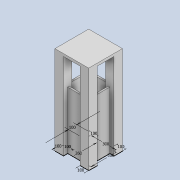
# Autodesk Inventor part: Part35
Saved by Autodesk Inventor 2021 (Build 250183000, 183)
## iProperties
Created: 2025-11-30
Part Number: Part35
Material: Generic
Document SubType Name: Modeling
Designer: huber
Density: 1 g/cm^3
Appearance: Default
Author: huber
Autodesk Inventor part; units mm, degrees
ref_plane "YZ Plane" through (0, 0, 0) normal (1, 0, 0) x (0, 1, 0)
ref_plane "XZ Plane" through (0, 0, 0) normal (0, 1, 0) x (-1, 0, 0)
ref_plane "XY Plane" through (0, 0, 0) normal (0, 0, 1) x (1, 0, 0)
sketch "Sketch1" plane through (0, 0, 0) normal (0, 1, 0) x (-1, 0, 0)
  line L0 (150, 150) -> (-150, 150)
  line L1 (-150, 150) -> (-150, -150)
  line L2 (-150, -150) -> (150, -150)
  line L3 (150, -150) -> (150, 150)
  line L4 (150, 150) -> (-150, -150) construction
  line L5 (-150, 150) -> (150, -150) construction
  line L6 (100, -100) -> (200, -100)
  line L7 (200, -100) -> (200, -200)
  line L8 (200, -200) -> (100, -200)
  line L9 (100, -200) -> (100, -100)
  line L10 (100, -100) -> (200, -200) construction
  line L11 (200, -100) -> (100, -200) construction
  line L12 (100, 200) -> (200, 200)
  line L13 (200, 200) -> (200, 100)
  line L14 (200, 100) -> (100, 100)
  line L15 (100, 100) -> (100, 200)
  line L16 (100, 200) -> (200, 100) construction
  line L17 (200, 200) -> (100, 100) construction
  line L18 (-100, 100) -> (-200, 100)
  line L19 (-200, 100) -> (-200, 200)
  line L20 (-200, 200) -> (-100, 200)
  line L21 (-100, 200) -> (-100, 100)
  line L22 (-100, 100) -> (-200, 200) construction
  line L23 (-200, 100) -> (-100, 200) construction
  line L24 (-100, -100) -> (-200, -100)
  line L25 (-200, -100) -> (-200, -200)
  line L26 (-200, -200) -> (-100, -200)
  line L27 (-100, -200) -> (-100, -100)
  line L28 (-100, -100) -> (-200, -200) construction
  line L29 (-200, -100) -> (-100, -200) construction
  line L30 (130, 130) -> (-130, 130)
  line L31 (-130, 130) -> (-130, -130)
  line L32 (-130, -130) -> (130, -130)
  line L33 (130, -130) -> (130, 130)
  line L34 (130, 130) -> (-130, -130) construction
  line L35 (-130, 130) -> (130, -130) construction
  point P0 (0, 0)
  dimension "d0" = 300
  dimension "d1" = 300
  dimension "d2" = 100
  dimension "d3" = 100
  dimension "d4" = 100
  dimension "d5" = 100
  dimension "d6" = 100
  dimension "d7" = 100
  dimension "d14" = 260
  constraints: 72 end point, 12 midpoint, 12 parallel, 6 horizontal, 6 perpendicular, 3 point on line
  measures "d0" distance of L1.end L2.end
  measures "d1" distance of L0.end L1.end
  measures "d2" distance of L7.end L8.end
  measures "d3" distance of L6.end L7.end
  measures "d4" distance of L12.end L13.end
  measures "d5" distance of L13.end L14.end
  measures "d6" distance of L19.end L20.end
  measures "d7" distance of L25.end L26.end
  measures "d14" distance between parallel lines of L30 L32
extrude "Extrusion1" add sketch "Sketch1" along normal blind 1050 contours L3 L14 L33 L30 L15 L0 | L0 L15 L12 L13 L14 L3 | L21 L30 L31 L18 L1 L0 | L0 L1 L18 L19 L20 L21 | L30 L33 L14 L15 | L6 L7 L8 L9 L2 L3 | L3 L2 L9 L32 L33 L6 | L21 L18 L31 L30 | L33 L32 L9 L6 | L24 L31 L32 L27 L2 L1 | L1 L2 L27 L26 L25 L24 | L24 L27 L32 L31
extrude "Extrusion2" add sketch "Sketch1" along normal blind 680 contours L3 L14 L33 L30 L15 L0 | L15 L30 L21 L0 | L3 L6 L33 L14 | L21 L30 L31 L18 L1 L0 | L3 L2 L9 L32 L33 L6 | L18 L31 L24 L1 | L2 L27 L32 L9 | L24 L31 L32 L27 L2 L1
sketch "Sketch2" plane through (0, 1050, 0) normal (0, 1, 0) x (1, 0, 0)
  line L0 (-200, -200) -> (-100, -200) projected
  line L1 (200, 100) -> (200, 200) projected
  line L2 (-200, -200) -> (200, -200)
  line L3 (200, -200) -> (200, 200)
  line L4 (200, 200) -> (-200, 200)
  line L5 (-200, 200) -> (-200, -200)
  point P0 (0, 0)
  constraints: 8 end point, 2 parallel, 1 horizontal, 1 perpendicular
extrude "Extrusion3" add sketch "Sketch2" against normal blind 30
extrude "Extrusion4" add sketch "Sketch1" along normal blind 10 contours L3 L14 L33 L30 L15 L0 | L15 L30 L21 L0 | L3 L6 L33 L14 | L21 L30 L31 L18 L1 L0 | L30 L33 L14 L15 | L15 L14 L33 L6 L9 L32 L27 L24 L31 L18 L21 L30 | L3 L2 L9 L32 L33 L6 | L21 L18 L31 L30 | L33 L32 L9 L6 | L18 L31 L24 L1 | L2 L27 L32 L9 | L24 L31 L32 L27 L2 L1 | L24 L27 L32 L31
body "Solid1"
